psu_support (Autodesk Fusion 360 design; units mm, degrees)
Autodesk Fusion 360 part; units mm, degrees
note: some values were not read from the file. Set by a fixed rule: which sketch regions a step uses.
sketch "Sketch1" plane through (0, 0, 0) normal (0, 1, 0) x (1, 0, 0)
  line L0 (0, 0) -> (0, 25)
  line L1 (0, 25) -> (3, 25)
  line L2 (3, 25) -> (3, 175.5)
  line L3 (3, 175.5) -> (88.5, 175.5)
  line L4 (88.5, 175.5) -> (88.5, 25)
  line L5 (88.5, 25) -> (30.5, 25)
  line L6 (30.5, 25) -> (30.5, 0)
  line L7 (30.5, 0) -> (34.5, 0)
  line L8 (34.5, 0) -> (34.5, 22)
  line L9 (34.5, 22) -> (91.5, 22)
  line L10 (91.5, 22) -> (91.5, 178.5)
  line L11 (91.5, 178.5) -> (0, 178.5)
  line L12 (0, 178.5) -> (0, 28)
  line L13 (0, 28) -> (-4, 28)
  line L14 (-4, 28) -> (-4, 0)
  line L15 (-4, 0) -> (0, 0)
  dimension "d1" = 4
  dimension "d2" = 3
  dimension "d3" = 3
  dimension "d4" = 3
  dimension "d5" = 3
  dimension "d6" = 3
  dimension "d7" = 4
  dimension "d8" = 85.5
  dimension "d9" = 150.5
  dimension "d10" = 25
  dimension "d11" = 25
  dimension "d12" = 3
  dimension "d13" = 30.5
  constraint vertical L0
  constraint perpendicular L0 L1
  constraint perpendicular L1 L2
  constraint perpendicular L0 L3
  constraint perpendicular L3 L4
  constraint perpendicular L4 L5
  constraint perpendicular L5 L6
  constraint perpendicular L6 L7
  constraint perpendicular L7 L8
  constraint perpendicular L8 L9
  constraint perpendicular L9 L10
  constraint perpendicular L10 L11
  constraint perpendicular L11 L12
  constraint perpendicular L12 L13
  constraint perpendicular L13 L14
  constraint horizontal L15
  constraint coincident L0.start L15.end
  constraint horizontal L1.end L5.end
  measures "d1" distance of L0 L14
  measures "d2" distance of L2 L12
  measures "d3" distance of L3 L11
  measures "d4" distance of L1 L13
  measures "d5" distance of L4 L10
  measures "d6" distance of L5 L9
  measures "d7" distance of L6 L8
  measures "d8" distance of L2.end L3.end
  measures "d9" distance of L3.end L4.end
  measures "d10" distance of L0.start L0.end
  measures "d11" distance of L5.end L6.end
  measures "d12" distance of L0.end L1.end
  measures "d13" distance of L0 L6
extrude "Extrude1" add sketch "Sketch1" along normal blind 4
sketch "Sketch2" plane through (-4, 0, 0) normal (-1, 0, 0) x (0, 0, 1)
  line L0 (-28, 0) -> (0, 0)
  line L1 (0, 0) -> (0, 4)
  line L2 (0, 4) -> (-28, 4)
  line L3 (-28, 4) -> (-28, 0)
  line L4 (-25, 0) -> (-25, 4)
  circle A0 centre (-10, 4) radius 1.6
  line L5 (0, 4) -> (-7.5, 8.3301)
  line L6 (-12.5, 8.3301) -> (-20, 4)
  arc A1 (-7.5, 8.3301) -> (-12.5, 8.3301) centre (-10, 4) ccw
  point P0 (-25, 2)
  dimension "d16" = 3.2
  dimension "d17" = 10
  dimension "d18" = 2
  dimension "d19" = 15
  dimension "d20" = 30
  constraint concentric A0 A1
  constraint midpoint L4 P0
  constraint coincident L1.end L2.start
  constraint tangent L5 A1
  constraint coincident L2 L6.end
  constraint tangent L6 A1
  measures "d16" diameter of A0
  measures "d17" diameter of A1
  measures "d18" vertical distance of A0.centre P0
  measures "d19" distance of L4 A0.centre
  measures "d20" angle of L2 L6
extrude "Extrude2" add sketch "Sketch2" against normal up to surface (4 mm away) contours L2 A0 L5 L6 A1
extrude "Extrude3" add sketch "Sketch2" against normal up to surface (4 mm away) from surface at -34.5 contours L2 A0 L5 L6 A1
extrude "Extrude4" cut sketch "Sketch2" against normal through all contours L2 A0 picked at (-9.8813, 3.48)
fillet "Fillet1" radius 3 12 edges at (-2, 4, -20) (32.5, 4, -20) (32.5, 4, 0) (32.5, 0, 0) (-2, 4, 0) (-2, 0, 0) (-4, 2, -28) (0, 2, -28) (0, 2, -178.5) (91.5, 2, -178.5) (91.5, 2, -22) (34.5, 2, -22)
equation "d2 = d4"
equation "d3 = d4"
equation "d5 = d4"
equation "d6 = d4"
